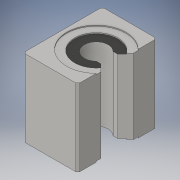
# Autodesk Inventor part: sbr12uu
Saved by Autodesk Inventor 2016 (Build 200138000, 138)
## iProperties
Created: 2016-06-30
Part Number: sbr12uu
Material: Generic
Document SubType Name: Modeling
Designer: brent
Density: 1 g/cm^3
Appearance: Default
Author: brent
Autodesk Inventor part; units mm, degrees
ref_plane "YZ Plane" through (0, 0, 0) normal (1, 0, 0) x (0, 1, 0)
ref_plane "XZ Plane" through (0, 0, 0) normal (0, 1, 0) x (-1, 0, 0)
ref_plane "XY Plane" through (0, 0, 0) normal (0, 0, 1) x (1, 0, 0)
sketch "Sketch1" plane through (0, 0, 0) normal (0, 1, 0) x (-1, 0, 0)
  circle A0 centre (0, 0) radius 6
  line L0 (17, 20) -> (-10.6, 20)
  line L1 (-10.6, 20) -> (-10.6, -20)
  line L2 (-10.6, -20) -> (17, -20)
  line L3 (17, -20) -> (17, 20)
  line L4 (0, 0) -> (17, 0) construction
  line L5 (-4.2353, 4.25) -> (-10.6, 4.25)
  line L6 (-10.6, 4.25) -> (-10.6, -4.25)
  line L7 (-10.6, -4.25) -> (-4.2353, -4.25)
  line L8 (-4.2353, -4.25) -> (-4.2353, 4.25)
  dimension "d0" = 12
  dimension "d1" = 27.6
  dimension "d2" = 40
  dimension "d3" = 17
  dimension "d4" = 8.5
  constraints: 18 end point, 4 parallel, 3 perpendicular, 2 horizontal, 2 point on circle, 1 centre point, 1 coincident, 1 midpoint, 1 point on line
  measures "d0" diameter of A0
  measures "d1" distance of L2.end L1.end
  measures "d2" distance of L2.end L0.start
  measures "d3" distance of L4.start L4.end
  measures "d4" distance of L7.end L5.start
extrude "Extrusion1" add sketch "Sketch1" along normal blind 39 contours A0 L5 L1 L0 L3 L2 L7
chamfer "Chamfer1" distance 4 angle 45 2 edges at (10.6, 19.5, 4.25) (10.6, 19.5, -4.25)
sketch "Sketch2" plane through (0, 39, 0) normal (0, 1, 0) x (1, 0, 0)
  arc A0 (4.2353, 4.25) -> (4.2353, -4.25) centre (0, 0) ccw projected
  circle A1 centre (0, 0) radius 11
  dimension "d10" = 22
  constraints: 1 centre point, 1 coincident
  measures "d10" diameter of A1
extrude "Extrusion2" cut sketch "Sketch2" against normal blind 1
sketch "Sketch3" plane through (0, 39, 0) normal (0, 1, 0) x (1, 0, 0)
  circle A0 centre (0, 0) radius 15
  dimension "d16" = 30
  constraints: 1 centre point, 1 coincident
  measures "d16" diameter of A0
extrude "Extrusion3" cut sketch "Sketch3" against normal blind 0.5
chamfer "Chamfer2" distance 1 angle 45 4 edges at (-17, 19.5, 20) (-17, 19.5, -20) (10.6, 19.5, -20) (10.6, 19.5, 20)
ref_plane "Work Plane1" through (0, 19.5, 0) normal (0, 1, 0) x (1, 0, 0)
mirror "Mirror1" about plane through (0, 19.5, 0) normal (0, 1, 0) of "Extrusion2", "Extrusion3"
sketch "Sketch4" plane through (-17, 0, -19) normal (-1, 0, 0) x (0, 0, 1)
  line L0 (0, 0) -> (0, 39) construction
  line L1 (0, 0) -> (38, 0) construction
  line L2 (38, 39) -> (38, 0) construction
  line L3 (0, 39) -> (38, 39) construction
  line L4 (0, 0) -> (0, 39) construction
  line L5 (0, 0) -> (38, 39) construction
  line L6 (33, 6.5) -> (5, 6.5) construction
  line L7 (5, 6.5) -> (5, 32.5) construction
  line L8 (5, 32.5) -> (33, 32.5) construction
  line L9 (33, 32.5) -> (33, 6.5) construction
  line L10 (33, 6.5) -> (5, 32.5) construction
  line L11 (5, 6.5) -> (33, 32.5) construction
  circle A0 centre (5, 6.5) radius 2
  circle A1 centre (33, 6.5) radius 2
  circle A2 centre (33, 32.5) radius 2
  circle A3 centre (5, 32.5) radius 2
  point P0 (19, 0)
  point P1 (19, 19.5)
  dimension "d19" = 28
  dimension "d20" = 26
  dimension "d21" = 4
  dimension "d22" = 4
  dimension "d23" = 4
  dimension "d24" = 4
  constraints: 14 end point, 4 centre point, 4 coincident, 3 midpoint, 2 parallel, 1 horizontal, 1 perpendicular
  measures "d19" distance of L7.end L8.end
  measures "d20" distance of L6.end L7.end
  measures "d21" diameter of A0
  measures "d22" diameter of A1
  measures "d23" diameter of A2
  measures "d24" diameter of A3
extrude "Extrusion4" cut sketch "Sketch4" against normal blind 10
thread "Thread1" size "M4x0.7" class "6H" standard "ISO Metric profile" full length
thread "Thread2" size "8-32 UNC" class "2B" standard "ANSI Unified Screw Threads" full length
thread "Thread3" size "8-32 UNC" class "2B" standard "ANSI Unified Screw Threads" full length
thread "Thread4" size "8-32 UNC" class "2B" standard "ANSI Unified Screw Threads" full length
body "Solid1"
